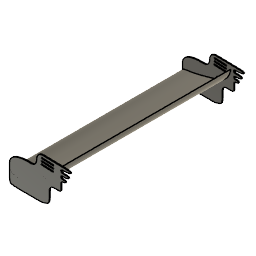
Airfoil_Design_Challenge_BITS (Autodesk Fusion 360 design; units mm, degrees)
Autodesk Fusion 360 part; units mm, degrees
(part 1 of 3)
sketch "Sketch2" plane through (0, 0, 0) normal (0, 1, 0) x (1, 0, 0)
  line L0 (0, 0) -> (212.4767, -57.0409) construction
  spline S0 degree 5 poles (212.4767, -57.0409) (212.4811, -57.0327) (212.4467, -56.9897) (212.2662, -56.8437) (211.8427, -56.5229) (211.2763, -56.0593) (210.7601, -55.5856) (210.2741, -55.0978) (209.7539, -54.5681) (209.168, -53.9856) (208.5221, -53.358) (207.8379, -52.7014) (207.1411, -52.0335) (206.4439, -51.3646) (205.7448, -50.6977) (205.0353, -50.0315) (204.304, -49.3629) (203.5422, -48.6889) (202.7475, -48.0094) (201.9215, -47.3254) (201.068, -46.6387) (200.192, -45.951) (199.2971, -45.2633) (198.3853, -44.5755) (197.4571, -43.8867) (196.5121, -43.1956) (195.5499, -42.5009) (194.5701, -41.8014) (193.573, -41.0967) (192.5596, -40.3867) (191.531, -39.6718) (190.4885, -38.9526) (189.4335, -38.2295) (188.367, -37.503) (187.2896, -36.7733) (186.2017, -36.0406) (185.1036, -35.3049) (183.9954, -34.5662) (182.8772, -33.8244) (181.7492, -33.0797) (180.6116, -32.3321) (179.4648, -31.5818) (178.3092, -30.8291) (177.1453, -30.0741) (175.9734, -29.3171) (174.7941, -28.5585) (173.6076, -27.7983) (172.4142, -27.037) (171.214, -26.2745) (170.0073, -25.5112) (168.7943, -24.7472) (167.575, -23.9826) (166.3497, -23.2178) (165.1186, -22.4528) (163.8818, -21.6879) (162.6396, -20.9232) (161.3921, -20.1589) (160.1396, -19.3954) (158.8823, -18.6326) (157.6203, -17.8709) (156.3539, -17.1105) (155.083, -16.3515) (153.808, -15.5943) (152.5288, -14.8389) (151.2457, -14.0856) (149.9587, -13.3347) (148.668, -12.5865) (147.3737, -11.8411) (146.076, -11.0988) (144.7749, -10.3599) (143.4707, -9.6246) (142.1634, -8.8933) (140.8531, -8.1661) (139.5399, -7.4433) (138.224, -6.725) (136.9055, -6.0116) (135.5843, -5.3032) (134.2607, -4.6001) (132.9347, -3.9025) (131.6065, -3.2107) (130.276, -2.5249) (128.9436, -1.8455) (127.6091, -1.1728) (126.2728, -0.5071) (124.9347, 0.1512) (123.5949, 0.8016) (122.2533, 1.4439) (120.9099, 2.0774) (119.5648, 2.7017) (118.2177, 3.3163) (116.8686, 3.9208) (115.5175, 4.5148) (114.1642, 5.0979) (112.8087, 5.6698) (111.4509, 6.2305) (110.0908, 6.7796) (108.7284, 7.3172) (107.3638, 7.8432) (105.9969, 8.3576) (104.6278, 8.8602) (103.2565, 9.3511) (101.8833, 9.83) (100.5082, 10.297) (99.1313, 10.7518) (97.7527, 11.1943) (96.3726, 11.6242) (94.991, 12.0415) (93.6081, 12.4458) (92.2239, 12.8369) (90.8384, 13.2148) (89.4519, 13.579) (88.0643, 13.9296) (86.6758, 14.2663) (85.2866, 14.5892) (83.8968, 14.8981) (82.5067, 15.1932) (81.1165, 15.4744) (79.7264, 15.7418) (78.3367, 15.9955) (76.9475, 16.2356) (75.5591, 16.4621) (74.1716, 16.6749) (72.7851, 16.8742) (71.4, 17.0599) (70.0162, 17.232) (68.6341, 17.3906) (67.2537, 17.5358) (65.8755, 17.6677) (64.4996, 17.7863) (63.1263, 17.8919) (61.7559, 17.9845) (60.3886, 18.0643) (59.0249, 18.1313) (57.6649, 18.1857) (56.309, 18.2276) (54.9573, 18.2569) (53.6102, 18.2736) (52.2679, 18.2779) (50.9307, 18.2696) (49.5988, 18.2488) (48.2726, 18.2154) (46.9524, 18.1694) (45.6385, 18.1109) (44.3312, 18.0398) (43.0308, 17.956) (41.7378, 17.8596) (40.4523, 17.7505) (39.1749, 17.6288) (37.9058, 17.4945) (36.6455, 17.3474) (35.3941, 17.1877) (34.1522, 17.0152) (32.92, 16.8299) (31.6978, 16.6317) (30.4861, 16.4207) (29.2853, 16.1966) (28.0958, 15.9595) (26.918, 15.7094) (25.7525, 15.4461) (24.5999, 15.1696) (23.4607, 14.8798) (22.3355, 14.5768) (21.2247, 14.2603) (20.1289, 13.9304) (19.0487, 13.587) (17.9846, 13.2299) (16.9373, 12.859) (15.9075, 12.4743) (14.896, 12.0756) (13.9038, 11.6629) (12.9318, 11.236) (11.9809, 10.7949) (11.052, 10.3396) (10.1459, 9.8701) (9.2635, 9.3866) (8.4059, 8.8889) (7.5744, 8.377) (6.7708, 7.8508) (5.9972, 7.3098) (5.2557, 6.754) (4.5484, 6.1836) (3.8771, 5.599) (3.2432, 5.0012) (2.6484, 4.3911) (2.0954, 3.7688) (1.5881, 3.1334) (1.1324, 2.4835) (0.7358, 1.8248) (0.4076, 1.1735) (0.1598, 0.566) (-0.0008, 0.0444) (-0.0815, -0.36) (-0.1201, -0.6567) (-0.145, -0.8932) (-0.1463, -1.2408) (-0.1178, -1.4667) (-0.1072, -1.5898) (-0.0507, -1.8099) (-0.0051, -1.9331) (0.0982, -2.1251) (0.1853, -2.2519) (0.289, -2.4175) (0.5475, -2.7065) (0.7064, -2.8823) (0.9696, -3.1172) (1.323, -3.4157) (1.6012, -3.648) (1.8666, -3.8408) (2.3156, -4.1171) (3.0047, -4.5094) (3.8866, -4.9842) (4.8656, -5.4778) (5.8455, -5.9275) (6.7856, -6.3085) (7.6894, -6.626) (8.585, -6.902) (9.5098, -7.1644) (10.4912, -7.4339) (11.5355, -7.7165) (12.6366, -8.0096) (13.7801, -8.3045) (14.9495, -8.591) (16.1317, -8.8613) (17.3214, -9.1127) (18.5188, -9.3462) (19.7275, -9.5655) (20.9531, -9.7752) (22.2012, -9.98) (23.475, -10.1832) (24.7753, -10.3861) (26.1011, -10.5891) (27.4501, -10.7914) (28.8195, -10.9921) (30.2063, -11.1904) (31.6084, -11.3859) (33.0247, -11.5791) (34.4546, -11.7708) (35.8983, -11.9624) (37.3562, -12.1554) (38.8286, -12.3512) (40.3159, -12.5513) (41.8181, -12.7565) (43.3347, -12.9675) (44.8651, -13.1845) (46.4085, -13.4076) (47.9638, -13.6368) (49.5301, -13.8718) (51.1066, -14.1126) (52.6927, -14.3591) (54.2877, -14.6112) (55.8914, -14.8691) (57.5035, -15.1329) (59.1238, -15.4028) (60.7521, -15.679) (62.3882, -15.962) (64.032, -16.2518) (65.6829, -16.5489) (67.3406, -16.8536) (69.0047, -17.166) (70.6745, -17.4866) (72.3495, -17.8154) (74.0292, -18.1525) (75.713, -18.498) (77.4005, -18.8518) (79.091, -19.2136) (80.7843, -19.5832) (82.4799, -19.9603) (84.1774, -20.3443) (85.8766, -20.7348) (87.5771, -21.1312) (89.2787, -21.5331) (90.9811, -21.94) (92.6841, -22.3512) (94.3874, -22.7663) (96.0908, -23.1849) (97.7942, -23.6065) (99.4973, -24.0306) (101.2001, -24.457) (102.9022, -24.8853) (104.6035, -25.3152) (106.3039, -25.7464) (108.0033, -26.1788) (109.7014, -26.6122) (111.398, -27.0465) (113.0931, -27.4815) (114.7865, -27.9172) (116.478, -28.3535) (118.1675, -28.7903) (119.8547, -29.2277) (121.5396, -29.6654) (123.2219, -30.1036) (124.9015, -30.5421) (126.5782, -30.981) (128.2518, -31.4202) (129.922, -31.8597) (131.5886, -32.2996) (133.2513, -32.7398) (134.9098, -33.1805) (136.5639, -33.6215) (138.2132, -34.063) (139.8575, -34.5051) (141.4964, -34.9476) (143.1296, -35.3908) (144.7568, -35.8345) (146.3777, -36.2789) (147.9922, -36.7238) (149.5999, -37.1693) (151.2005, -37.6154) (152.7937, -38.0619) (154.3793, -38.5087) (155.9568, -38.9557) (157.5259, -39.4027) (159.0863, -39.8495) (160.6374, -40.2958) (162.179, -40.7415) (163.7106, -41.1863) (165.232, -41.63) (166.7429, -42.0726) (168.2431, -42.514) (169.7326, -42.9541) (171.2113, -43.3932) (172.6792, -43.8311) (174.136, -44.268) (175.5817, -44.7038) (177.0156, -45.1382) (178.4372, -45.5712) (179.8454, -46.0021) (181.2394, -46.4304) (182.6181, -46.8558) (183.9806, -47.2777) (185.3264, -47.6961) (186.6553, -48.1109) (187.9678, -48.5227) (189.2648, -48.9323) (190.5471, -49.3404) (191.8152, -49.7475) (193.069, -50.1538) (194.3073, -50.5586) (195.5275, -50.9603) (196.7252, -51.3563) (197.8965, -51.744) (199.0375, -52.1213) (200.1469, -52.4876) (201.2255, -52.8442) (202.2787, -53.1956) (203.3138, -53.5477) (204.3365, -53.9054) (205.3477, -54.2702) (206.3402, -54.6382) (207.2946, -54.9968) (208.1849, -55.3291) (208.9927, -55.6238) (209.7156, -55.8811) (210.3847, -56.1254) (211.0537, -56.3976) (211.7317, -56.7089) (212.2101, -56.9445) (212.4199, -57.0387) (212.4722, -57.049) (212.4767, -57.0409) knots 0 0 0 0 0 0 0.0028169 0.0056338 0.0084507 0.01126761 0.01408451 0.01690141 0.01971831 0.02253521 0.02535211 0.02816901 0.03098592 0.03380282 0.03661972 0.03943662 0.04225352 0.04507042 0.04788732 0.05070423 0.05352113 0.05633803 0.05915493 0.06197183 0.06478873 0.06760563 0.07042254 0.07323944 0.07605634 0.07887324 0.08169014 0.08450704 0.08732394 0.09014085 0.09295775 0.09577465 0.09859155 0.10140845 0.10422535 0.10704225 0.10985915 0.11267606 0.11549296 0.11830986 0.12112676 0.12394366 0.12676056 0.12957746 0.13239437 0.13521127 0.13802817 0.14084507 0.14366197 0.14647887 0.14929577 0.15211268 0.15492958 0.15774648 0.16056338 0.16338028 0.16619718 0.16901408 0.17183099 0.17464789 0.17746479 0.18028169 0.18309859 0.18591549 0.18873239 0.1915493 0.1943662 0.1971831 0.2 0.2028169 0.2056338 0.2084507 0.21126761 0.21408451 0.21690141 0.21971831 0.22253521 0.22535211 0.22816901 0.23098592 0.23380282 0.23661972 0.23943662 0.24225352 0.24507042 0.24788732 0.25070423 0.25352113 0.25633803 0.25915493 0.26197183 0.26478873 0.26760563 0.27042254 0.27323944 0.27605634 0.27887324 0.28169014 0.28450704 0.28732394 0.29014085 0.29295775 0.29577465 0.29859155 0.30140845 0.30422535 0.30704225 0.30985915 0.31267606 0.31549296 0.31830986 0.32112676 0.32394366 0.32676056 0.32957746 0.33239437 0.33521127 0.33802817 0.34084507 0.34366197 0.34647887 0.34929577 0.35211268 0.35492958 0.35774648 0.36056338 0.36338028 0.36619718 0.36901408 0.37183099 0.37464789 0.37746479 0.38028169 0.38309859 0.38591549 0.38873239 0.3915493 0.3943662 0.3971831 0.4 0.4028169 0.4056338 0.4084507 0.41126761 0.41408451 0.41690141 0.41971831 0.42253521 0.42535211 0.42816901 0.43098592 0.43380282 0.43661972 0.43943662 0.44225352 0.44507042 0.44788732 0.45070423 0.45352113 0.45633803 0.45915493 0.46197183 0.46478873 0.46760563 0.47042254 0.47323944 0.47605634 0.47887324 0.48169014 0.48450704 0.48732394 0.49014085 0.49295775 0.49577465 0.49859155 0.50140845 0.50422535 0.50704225 0.50985915 0.51267606 0.51549296 0.51830986 0.52112676 0.52394366 0.52676056 0.52957746 0.53239437 0.53521127 0.53802817 0.54084507 0.54366197 0.54647887 0.54929577 0.55211268 0.55492958 0.55774648 0.56056338 0.56338028 0.56619718 0.56901408 0.57183099 0.57464789 0.57746479 0.58028169 0.58309859 0.58591549 0.58873239 0.5915493 0.5943662 0.5971831 0.6 0.6028169 0.6056338 0.6084507 0.61126761 0.61408451 0.61690141 0.61971831 0.62253521 0.62535211 0.62816901 0.63098592 0.63380282 0.63661972 0.63943662 0.64225352 0.64507042 0.64788732 0.65070423 0.65352113 0.65633803 0.65915493 0.66197183 0.66478873 0.66760563 0.67042254 0.67323944 0.67605634 0.67887324 0.68169014 0.68450704 0.68732394 0.69014085 0.69295775 0.69577465 0.69859155 0.70140845 0.70422535 0.70704225 0.70985915 0.71267606 0.71549296 0.71830986 0.72112676 0.72394366 0.72676056 0.72957746 0.73239437 0.73521127 0.73802817 0.74084507 0.74366197 0.74647887 0.74929577 0.75211268 0.75492958 0.75774648 0.76056338 0.76338028 0.76619718 0.76901408 0.77183099 0.77464789 0.77746479 0.78028169 0.78309859 0.78591549 0.78873239 0.7915493 0.7943662 0.7971831 0.8 0.8028169 0.8056338 0.8084507 0.81126761 0.81408451 0.81690141 0.81971831 0.82253521 0.82535211 0.82816901 0.83098592 0.83380282 0.83661972 0.83943662 0.84225352 0.84507042 0.84788732 0.85070423 0.85352113 0.85633803 0.85915493 0.86197183 0.86478873 0.86760563 0.87042254 0.87323944 0.87605634 0.87887324 0.88169014 0.88450704 0.88732394 0.89014085 0.89295775 0.89577465 0.89859155 0.90140845 0.90422535 0.90704225 0.90985915 0.91267606 0.91549296 0.91830986 0.92112676 0.92394366 0.92676056 0.92957746 0.93239437 0.93521127 0.93802817 0.94084507 0.94366197 0.94647887 0.94929577 0.95211268 0.95492958 0.95774648 0.96056338 0.96338028 0.96619718 0.96901408 0.97183099 0.97464789 0.97746479 0.98028169 0.98309859 0.98591549 0.98873239 0.9915493 0.9943662 0.9971831 1 1 1 1 1 1
  line L1 (212.4767, -57.0409) -> (212.4767, -65.0409) construction
  line L2 (212.4767, -65.0409) -> (207.4767, -65.0409) construction
  line L3 (207.4767, -65.0409) -> (293.6674, -148.5343) construction
  spline S1 degree 5 poles (293.6674, -148.5343) (293.6768, -148.4864) (293.6956, -148.3905) (293.7231, -148.2462) (293.7587, -148.0528) (293.8015, -147.8097) (293.8425, -147.5655) (293.8817, -147.321) (293.919, -147.0771) (293.9544, -146.8358) (293.9879, -146.5991) (294.0191, -146.3692) (294.0478, -146.1475) (294.0735, -145.9347) (294.0954, -145.7298) (294.1126, -145.5303) (294.1241, -145.3328) (294.1293, -145.1341) (294.128, -144.9318) (294.1207, -144.7252) (294.1085, -144.5151) (294.093, -144.3031) (294.0755, -144.0911) (294.0574, -143.8807) (294.0397, -143.6731) (294.0228, -143.4686) (294.007, -143.2671) (293.9917, -143.0681) (293.976, -142.8708) (293.9584, -142.674) (293.9376, -142.4768) (293.9125, -142.2784) (293.8827, -142.0782) (293.8491, -141.8763) (293.8131, -141.6731) (293.7762, -141.4693) (293.7399, -141.2654) (293.7045, -141.0618) (293.6698, -140.8583) (293.635, -140.6548) (293.5992, -140.4513) (293.5615, -140.2476) (293.5218, -140.044) (293.4801, -139.8409) (293.437, -139.6388) (293.3934, -139.4383) (293.3501, -139.2401) (293.3083, -139.0447) (293.2688, -138.8526) (293.2322, -138.6639) (293.1987, -138.4787) (293.1676, -138.2963) (293.138, -138.116) (293.1084, -137.9368) (293.0773, -137.7575) (293.0435, -137.577) (293.0057, -137.3943) (292.9634, -137.2086) (292.9165, -137.0197) (292.8656, -136.8278) (292.812, -136.6337) (292.7573, -136.4384) (292.7032, -136.2432) (292.6508, -136.0487) (292.6006, -135.8552) (292.5524, -135.6626) (292.5058, -135.4705) (292.4599, -135.2784) (292.4141, -135.0858) (292.3676, -134.8923) (292.3198, -134.6977) (292.2703, -134.5018) (292.2189, -134.3047) (292.1654, -134.1061) (292.1102, -133.9064) (292.0535, -133.7056) (291.9957, -133.504) (291.9372, -133.3019) (291.8786, -133.0998) (291.8202, -132.898) (291.7624, -132.6969) (291.7053, -132.4967) (291.6489, -132.2975) (291.593, -132.0993) (291.5373, -131.902) (291.4815, -131.7052) (291.4251, -131.5087) (291.368, -131.3122) (291.3097, -131.1154) (291.2502, -130.9181) (291.1895, -130.7202) (291.1276, -130.5216) (291.0648, -130.3225) (291.0015, -130.1231) (290.938, -129.9237) (290.8745, -129.7244) (290.8114, -129.5255) (290.7487, -129.3268) (290.6864, -129.1284) (290.6243, -128.9301) (290.5624, -128.7318) (290.5002, -128.5334) (290.4376, -128.3347) (290.3743, -128.1355) (290.31, -127.9358) (290.2447, -127.7355) (290.1784, -127.5346) (290.1113, -127.3332) (290.0434, -127.1314) (289.9749, -126.9291) (289.9058, -126.7263) (289.8362, -126.523) (289.766, -126.3193) (289.6952, -126.1149) (289.6237, -125.91) (289.5515, -125.7046) (289.4786, -125.4988) (289.4049, -125.2925) (289.3305, -125.0859) (289.2555, -124.879) (289.1798, -124.6716) (289.1035, -124.4638) (289.0266, -124.2553) (288.9491, -124.0462) (288.8709, -123.8365) (288.7921, -123.6263) (288.7126, -123.4158) (288.6325, -123.2054) (288.5517, -122.9951) (288.4706, -122.7851) (288.3893, -122.5756) (288.3084, -122.3664) (288.228, -122.1576) (288.1482, -121.949) (288.069, -121.7404) (287.9898, -121.5316) (287.9099, -121.3224) (287.8287, -121.1126) (287.7458, -120.902) (287.6607, -120.6905) (287.5738, -120.4782) (287.4854, -120.2651) (287.3962, -120.0512) (287.3067, -119.8367) (287.2173, -119.6217) (287.1282, -119.4062) (287.0391, -119.1904) (286.9498, -118.9742) (286.86, -118.7578) (286.7693, -118.5411) (286.6776, -118.3242) (286.5848, -118.1069) (286.4909, -117.8894) (286.3959, -117.6716) (286.3001, -117.4534) (286.2035, -117.235) (286.1065, -117.0164) (286.0092, -116.7976) (285.9116, -116.5786) (285.8139, -116.3594) (285.7159, -116.1401) (285.6173, -115.9203) (285.5177, -115.7) (285.417, -115.4789) (285.3146, -115.257) (285.2107, -115.0343) (285.1053, -114.8107) (284.9989, -114.5866) (284.8919, -114.3621) (284.7847, -114.1374) (284.6779, -113.9129) (284.5716, -113.6886) (284.4657, -113.4646) (284.3599, -113.2408) (284.254, -113.017) (284.1475, -112.7932) (284.0402, -112.5692) (283.9317, -112.3449) (283.8221, -112.1202) (283.7113, -111.895) (283.5995, -111.6695) (283.4868, -111.4436) (283.3734, -111.2175) (283.2596, -110.9912) (283.1454, -110.765) (283.0311, -110.539) (282.9167, -110.3134) (282.8023, -110.0881) (282.6877, -109.8632) (282.5728, -109.6386) (282.4573, -109.4141) (282.341, -109.1897) (282.2237, -108.9651) (282.1053, -108.7403) (281.9857, -108.5153) (281.8652, -108.2903) (281.7439, -108.0653) (281.6219, -107.8405) (281.4996, -107.6161) (281.377, -107.3922) (281.2542, -107.1688) (281.1312, -106.9459) (281.0078, -106.7234) (280.8841, -106.5012) (280.76, -106.2793) (280.6355, -106.0577) (280.5104, -105.8363) (280.3849, -105.6151) (280.259, -105.3941) (280.1327, -105.1735) (280.006, -104.9531) (279.8791, -104.7331) (279.7518, -104.5133) (279.6242, -104.2939) (279.4963, -104.0747) (279.3681, -103.8557) (279.2396, -103.637) (279.1107, -103.4185) (278.9817, -103.2002) (278.8523, -102.9821) (278.7227, -102.7641) (278.5929, -102.5464) (278.4627, -102.3289) (278.3322, -102.1117) (278.2013, -101.8948) (278.0699, -101.6783) (277.9379, -101.4623) (277.8053, -101.2469) (277.672, -101.0319) (277.5381, -100.8175) (277.4034, -100.6036) (277.2682, -100.3902) (277.1323, -100.1774) (276.9957, -99.965) (276.8586, -99.7532) (276.7208, -99.5419) (276.5825, -99.331) (276.4435, -99.1207) (276.304, -98.9108) (276.1641, -98.7013) (276.0238, -98.4921) (275.8833, -98.2831) (275.7426, -98.0742) (275.6018, -97.8654) (275.461, -97.6565) (275.3202, -97.4478) (275.1793, -97.2391) (275.0382, -97.0305) (274.897, -96.8221) (274.7554, -96.6139) (274.6134, -96.4061) (274.4711, -96.1986) (274.3283, -95.9914) (274.1851, -95.7847) (274.0415, -95.5782) (273.8974, -95.3722) (273.7529, -95.1666) (273.6079, -94.9613) (273.4623, -94.7566) (273.3161, -94.5524) (273.1693, -94.3487) (273.0219, -94.1455) (272.8739, -93.9428) (272.7253, -93.7407) (272.5762, -93.539) (272.4265, -93.3378) (272.2764, -93.137) (272.1258, -92.9365) (271.9748, -92.7365) (271.8234, -92.5368) (271.6715, -92.3375) (271.5192, -92.1387) (271.3664, -91.9403) (271.2131, -91.7423) (271.0593, -91.5448) (270.905, -91.3477) (270.7502, -91.151) (270.5949, -90.9547) (270.4391, -90.7588) (270.2828, -90.5633) (270.1261, -90.3683) (269.9689, -90.1736) (269.8113, -89.9794) (269.6533, -89.7855) (269.495, -89.592) (269.3364, -89.3989) (269.1774, -89.206) (269.0183, -89.0134) (268.8588, -88.821) (268.699, -88.6289) (268.539, -88.437) (268.3786, -88.2455) (268.2177, -88.0543) (268.0564, -87.8636) (267.8947, -87.6734) (267.7323, -87.4836) (267.5695, -87.2944) (267.4061, -87.1057) (267.2421, -86.9175) (267.0776, -86.7297) (266.9126, -86.5424) (266.747, -86.3556) (266.5809, -86.1692) (266.4144, -85.9833) (266.2473, -85.7978) (266.0798, -85.6129) (265.9118, -85.4284) (265.7434, -85.2445) (265.5744, -85.0611) (265.405, -84.8782) (265.2351, -84.6958) (265.0647, -84.5138) (264.8938, -84.3324) (264.7224, -84.1513) (264.5506, -83.9707) (264.3783, -83.7904) (264.2056, -83.6106) (264.0325, -83.4311) (263.8588, -83.252) (263.6848, -83.0735) (263.5102, -82.8954) (263.3351, -82.7179) (263.1595, -82.541) (262.9834, -82.3648) (262.8066, -82.1891) (262.6292, -82.0141) (262.4512, -81.8398) (262.2725, -81.666) (262.0931, -81.4928) (261.9132, -81.3202) (261.7327, -81.1482) (261.5516, -80.9767) (261.37, -80.8059) (261.1879, -80.6356) (261.0053, -80.4659) (260.8221, -80.2969) (260.6384, -80.1284) (260.4541, -79.9606) (260.2692, -79.7934) (260.0837, -79.6268) (259.8976, -79.4607) (259.7111, -79.295) (259.5241, -79.1298) (259.3367, -78.965) (259.149, -78.8006) (258.9609, -78.6365) (258.7724, -78.4729) (258.5835, -78.3099) (258.3939, -78.1475) (258.2038, -77.9859) (258.013, -77.825) (257.8216, -77.6649) (257.6296, -77.5054) (257.4371, -77.3465) (257.2441, -77.188) (257.0507, -77.03) (256.857, -76.8723) (256.6629, -76.715) (256.4684, -76.5581) (256.2734, -76.4017) (256.078, -76.2458) (255.882, -76.0904) (255.6856, -75.9356) (255.4888, -75.7814) (255.2915, -75.6276) (255.0939, -75.4743) (254.896, -75.3214) (254.6978, -75.1689) (254.4992, -75.0167) (254.3003, -74.865) (254.1011, -74.7138) (253.9013, -74.563) (253.7011, -74.4128) (253.5004, -74.2631) (253.2991, -74.114) (253.0973, -73.9654) (252.895, -73.8174) (252.6923, -73.67) (252.4891, -73.5231) (252.2854, -73.3769) (252.0812, -73.2312) (251.8765, -73.0861) (251.6714, -72.9415) (251.4657, -72.7976) (251.2596, -72.6543) (251.0529, -72.5116) (250.8457, -72.3696) (250.6379, -72.2282) (250.4296, -72.0875) (250.2207, -71.9475) (250.0113, -71.8081) (249.8014, -71.6694) (249.591, -71.5313) (249.3801, -71.3938) (249.1687, -71.2569) (248.9569, -71.1206) (248.7445, -70.9849) (248.5316, -70.8498) (248.3182, -70.7155) (248.1042, -70.5818) (247.8897, -70.4489) (247.6747, -70.3166) (247.4592, -70.1849) (247.2432, -70.0537) (247.0269, -69.9231) (246.8103, -69.7928) (246.5933, -69.663) (246.3759, -69.5337) (246.1581, -69.405) (245.9398, -69.2769) (245.7209, -69.1496) (245.5014, -69.0231) (245.2812, -68.8974) (245.0605, -68.7725) (244.8392, -68.6483) (244.6174, -68.5248) (244.3952, -68.4019) (244.1725, -68.2796) (243.9494, -68.1579) (243.7259, -68.0368) (243.5018, -67.9165) (243.2771, -67.7968) (243.0517, -67.678) (242.8256, -67.5602) (242.5988, -67.4432) (242.3714, -67.3272) (242.1435, -67.212) (241.9151, -67.0977) (241.6862, -66.9842) (241.4569, -66.8714) (241.2271, -66.7591) (240.9968, -66.6473) (240.7659, -66.5359) (240.5343, -66.4248) (240.3021, -66.3142) (240.0694, -66.2041) (239.8364, -66.0947) (239.6032, -65.9864) (239.3702, -65.8792) (239.1374, -65.7735) (238.9053, -65.6693) (238.6737, -65.5665) (238.443, -65.4651) (238.2131, -65.3648) (237.984, -65.2656) (237.756, -65.1674) (237.529, -65.0703) (237.3033, -64.9748) (237.0791, -64.8811) (236.8564, -64.7896) (236.6354, -64.7008) (236.4161, -64.6146) (236.1985, -64.531) (235.9825, -64.4498) (235.7678, -64.3704) (235.5542, -64.2925) (235.3415, -64.2156) (235.1294, -64.1395) (234.9177, -64.064) (234.7062, -63.9892) (234.4949, -63.9151) (234.2838, -63.8418) (234.0728, -63.7694) (233.8622, -63.6979) (233.6522, -63.6276) (233.4431, -63.5585) (233.235, -63.4907) (233.028, -63.4243) (232.8222, -63.3596) (232.6176, -63.2964) (232.4141, -63.235) (232.2116, -63.1753) (232.0101, -63.117) (231.8095, -63.0601) (231.6095, -63.0043) (231.4102, -62.9493) (231.2114, -62.8948) (231.0131, -62.8404) (230.8151, -62.786) (230.6174, -62.7315) (230.4202, -62.6773) (230.2237, -62.6237) (230.028, -62.5718) (229.8335, -62.5222) (229.6403, -62.4756) (229.4483, -62.4318) (229.2571, -62.3902) (229.0665, -62.3499) (228.8759, -62.3096) (228.6851, -62.2686) (228.4939, -62.2268) (228.3025, -62.1845) (228.1113, -62.1424) (227.9205, -62.1012) (227.7304, -62.0617) (227.5411, -62.024) (227.3528, -61.9882) (227.1654, -61.9541) (226.9787, -61.9214) (226.7925, -61.8895) (226.6064, -61.8578) (226.4202, -61.8259) (226.2337, -61.7936) (226.0468, -61.761) (225.8598, -61.7288) (225.6729, -61.6976) (225.4864, -61.668) (225.3005, -61.6404) (225.1153, -61.6152) (224.931, -61.5922) (224.7475, -61.5712) (224.5646, -61.5517) (224.382, -61.533) (224.1994, -61.5145) (224.0165, -61.4957) (223.8333, -61.4764) (223.6499, -61.4569) (223.4666, -61.4377) (223.2838, -61.4192) (223.1021, -61.4018) (222.9218, -61.3856) (222.7434, -61.3706) (222.5671, -61.3569) (222.3932, -61.3447) (222.2216, -61.3344) (222.0522, -61.3265) (221.8843, -61.321) (221.7174, -61.3174) (221.5506, -61.3143) (221.3829, -61.3103) (221.2139, -61.304) (221.0433, -61.2952) (220.8716, -61.2847) (220.6996, -61.2738) (220.5283, -61.2642) (220.3584, -61.2574) (220.1906, -61.2545) (220.0253, -61.2561) (219.8625, -61.2618) (219.7019, -61.2701) (219.5426, -61.2788) (219.3838, -61.286) (219.225, -61.2911) (219.0656, -61.2949) (218.9057, -61.2989) (218.7451, -61.3043) (218.5842, -61.3117) (218.4233, -61.3205) (218.2626, -61.3297) (218.1019, -61.3387) (217.9411, -61.3473) (217.7796, -61.3561) (217.6171, -61.3655) (217.4538, -61.3758) (217.2905, -61.3871) (217.128, -61.3995) (216.9672, -61.4129) (216.8082, -61.428) (216.6511, -61.4451) (216.4953, -61.4648) (216.3406, -61.4868) (216.1865, -61.51) (216.0328, -61.5334) (215.8792, -61.5559) (215.7256, -61.5777) (215.5716, -61.5998) (215.4172, -61.6232) (215.2621, -61.6487) (215.1063, -61.6757) (214.9498, -61.7034) (214.7928, -61.731) (214.6356, -61.7583) (214.4788, -61.786) (214.3228, -61.815) (214.1682, -61.846) (214.0153, -61.8796) (213.8644, -61.9156) (213.7155, -61.9537) (213.5684, -61.9931) (213.4224, -62.033) (213.277, -62.0726) (213.1313, -62.1114) (212.9852, -62.1493) (212.8384, -62.1867) (212.6912, -62.2241) (212.5441, -62.2616) (212.398, -62.2998) (212.2537, -62.3389) (212.1118, -62.3794) (211.9722, -62.4221) (211.8346, -62.4676) (211.6985, -62.5164) (211.5633, -62.568) (211.4284, -62.6218) (211.2932, -62.6766) (211.157, -62.7316) (211.0193, -62.7859) (210.8798, -62.8396) (210.7392, -62.894) (210.5993, -62.9518) (210.4613, -63.0152) (210.3258, -63.0848) (210.1913, -63.1581) (210.0554, -63.2311) (209.916, -63.3002) (209.773, -63.3649) (209.6282, -63.428) (209.4841, -63.4934) (209.3426, -63.5641) (209.2034, -63.6398) (209.0654, -63.7186) (208.9272, -63.7981) (208.7894, -63.8774) (208.6546, -63.9579) (208.5258, -64.0418) (208.4054, -64.1312) (208.2938, -64.227) (208.1892, -64.3286) (208.089, -64.4344) (207.99, -64.5411) (207.8892, -64.6451) (207.7852, -64.744) (207.6789, -64.8386) (207.5744, -64.9339) (207.4764, -65.0358) (207.3881, -65.1484) (207.3093, -65.2708) (207.2384, -65.4001) (207.1749, -65.5326) (207.1218, -65.6678) (207.0847, -65.8067) (207.0685, -65.9497) (207.0749, -66.0939) (207.1017, -66.2337) (207.1462, -66.3645) (207.2086, -66.4863) (207.2932, -66.6055) (207.4049, -66.7308) (207.5469, -66.8691) (207.7174, -67.0225) (207.911, -67.1883) (208.1201, -67.3615) (208.3363, -67.5358) (208.5523, -67.7052) (208.7635, -67.8661) (208.9687, -68.0175) (209.1688, -68.1608) (209.3666, -68.2982) (209.5652, -68.4326) (209.7673, -68.5666) (209.9742, -68.7015) (210.1861, -68.8373) (210.402, -68.9736) (210.6206, -69.1092) (210.8404, -69.243) (211.0603, -69.3743) (211.2799, -69.5027) (211.4994, -69.6285) (211.7189, -69.7522) (211.9392, -69.8742) (212.1608, -69.9951) (212.3839, -70.1152) (212.6087, -70.2344) (212.8349, -70.3527) (213.0623, -70.4699) (213.2907, -70.5857) (213.5198, -70.6999) (213.7495, -70.8127) (213.9797, -70.9244) (214.2104, -71.0351) (214.4418, -71.1453) (214.6737, -71.2551) (214.9062, -71.3648) (215.1392, -71.4742) (215.3725, -71.5831) (215.6059, -71.6912) (215.8391, -71.7983) (216.0718, -71.9039) (216.304, -72.0078) (216.5355, -72.1101) (216.7662, -72.2106) (216.996, -72.3096) (217.225, -72.4071) (217.4532, -72.5034) (217.6809, -72.5988) (217.908, -72.6934) (218.1348, -72.7876) (218.3614, -72.8815) (218.5878, -72.9752) (218.8141, -73.0687) (219.0401, -73.1616) (219.2656, -73.2537) (219.4905, -73.3447) (219.7146, -73.4343) (219.9379, -73.5225) (220.1602, -73.6091) (220.3817, -73.6946) (220.6025, -73.7791) (220.8229, -73.8629) (221.0428, -73.9463) (221.2625, -74.0296) (221.4819, -74.1126) (221.701, -74.1955) (221.9198, -74.278) (222.1382, -74.3601) (222.3562, -74.4417) (222.5735, -74.5226) (222.7903, -74.6029) (223.0064, -74.6825) (223.2218, -74.7614) (223.4366, -74.8399) (223.6509, -74.9179) (223.8649, -74.9956) (224.0788, -75.0731) (224.2926, -75.1507) (224.5065, -75.2283) (224.7206, -75.3062) (224.9347, -75.3843) (225.1489, -75.4626) (225.363, -75.5412) (225.577, -75.6198) (225.791, -75.6985) (226.0049, -75.7769) (226.2188, -75.855) (226.4328, -75.9328) (226.6468, -76.0102) (226.861, -76.0875) (227.0752, -76.1651) (227.2895, -76.2431) (227.5037, -76.3219) (227.7177, -76.4015) (227.9315, -76.4815) (228.145, -76.5617) (228.3579, -76.6414) (228.5703, -76.7203) (228.7821, -76.798) (228.9934, -76.8746) (229.2042, -76.9506) (229.4147, -77.0265) (229.625, -77.1028) (229.8353, -77.1797) (230.0456, -77.2574) (230.2559, -77.3354) (230.4662, -77.4134) (230.6765, -77.4909) (230.8868, -77.5676) (231.0972, -77.6438) (231.3078, -77.7196) (231.5187, -77.7958) (231.73, -77.8728) (231.9417, -77.951) (232.1539, -78.0305) (232.3664, -78.1112) (232.5793, -78.1925) (232.7922, -78.274) (233.0052, -78.3555) (233.2181, -78.4365) (233.4308, -78.517) (233.6433, -78.5971) (233.8556, -78.6769) (234.0676, -78.7567) (234.2796, -78.8367) (234.4915, -78.9171) (234.7037, -78.9982) (234.9161, -79.08) (235.1289, -79.1627) (235.3422, -79.2462) (235.556, -79.3306) (235.7702, -79.4156) (235.9847, -79.5011) (236.1996, -79.5871) (236.4148, -79.6735) (236.6304, -79.7605) (236.8464, -79.8482) (237.0628, -79.9367) (237.2797, -80.0261) (237.4971, -80.1164) (237.7148, -80.2073) (237.9327, -80.2987) (238.1507, -80.3901) (238.3686, -80.4813) (238.5865, -80.5722) (238.8042, -80.6629) (239.022, -80.7535) (239.2397, -80.8443) (239.4577, -80.9357) (239.6759, -81.0279) (239.8945, -81.1211) (240.1134, -81.2154) (240.3326, -81.3109) (240.5522, -81.4073) (240.7719, -81.5047) (240.9919, -81.6027) (241.212, -81.7014) (241.4323, -81.8006) (241.6528, -81.9001) (241.8735, -82) (242.0944, -82.1002) (242.3157, -82.201) (242.5373, -82.3024) (242.7595, -82.4048) (242.9822, -82.5084) (243.2056, -82.6132) (243.4297, -82.7194) (243.6544, -82.8269) (243.8798, -82.9356) (244.1059, -83.0452) (244.3324, -83.1556) (244.5594, -83.2665) (244.7866, -83.3778) (245.0138, -83.4892) (245.241, -83.6007) (245.4679, -83.7123) (245.6943, -83.8239) (245.9204, -83.9357) (246.1462, -84.0478) (246.3717, -84.1606) (246.5972, -84.2741) (246.8227, -84.3885) (247.0484, -84.5041) (247.2742, -84.6208) (247.5002, -84.7386) (247.7261, -84.8572) (247.9519, -84.9764) (248.1773, -85.0961) (248.4023, -85.2161) (248.6268, -85.3364) (248.8509, -85.4568) (249.0745, -85.5776) (249.2978, -85.6986) (249.5208, -85.82) (249.7436, -85.9418) (249.9662, -86.0641) (250.1886, -86.1868) (250.4107, -86.31) (250.6326, -86.4336) (250.8542, -86.5577) (251.0755, -86.6821) (251.2964, -86.807) (251.517, -86.9323) (251.7373, -87.0579) (251.9571, -87.184) (252.1766, -87.3106) (252.3957, -87.4377) (252.6144, -87.5653) (252.8327, -87.6934) (253.0504, -87.8222) (253.2678, -87.9515) (253.4847, -88.0814) (253.7011, -88.2119) (253.9171, -88.3429) (254.1328, -88.4745) (254.3481, -88.6065) (254.563, -88.739) (254.7775, -88.8719) (254.9916, -89.0054) (255.2052, -89.1395) (255.4184, -89.2741) (255.6311, -89.4094) (255.8433, -89.5453) (256.055, -89.6818) (256.2664, -89.8187) (256.4775, -89.9559) (256.6884, -90.0934) (256.8992, -90.2311) (257.1098, -90.3689) (257.3202, -90.507) (257.5304, -90.6455) (257.7402, -90.7843) (257.9496, -90.9237) (258.1585, -91.0637) (258.3669, -91.2042) (258.5748, -91.3454) (258.7823, -91.4871) (258.9894, -91.6294) (259.1961, -91.772) (259.4025, -91.915) (259.6086, -92.0585) (259.8142, -92.2023) (260.0195, -92.3467) (260.2244, -92.4916) (260.4287, -92.637) (260.6326, -92.7831) (260.836, -92.9298) (261.0388, -93.077) (261.2412, -93.2249) (261.4431, -93.3732) (261.6446, -93.5221) (261.8457, -93.6714) (262.0463, -93.8213) (262.2466, -93.9716) (262.4464, -94.1224) (262.6458, -94.2737) (262.8449, -94.4254) (263.0435, -94.5777) (263.2416, -94.7304) (263.4394, -94.8836) (263.6367, -95.0373) (263.8336, -95.1915) (264.0301, -95.3461) (264.2261, -95.5013) (264.4216, -95.657) (264.6167, -95.8133) (264.8113, -95.97) (265.0055, -96.1273) (265.1992, -96.2851) (265.3925, -96.4433) (265.5854, -96.6021) (265.7778, -96.7613) (265.9698, -96.9209) (266.1614, -97.0811) (266.3525, -97.2417) (266.5431, -97.4029) (266.7332, -97.5647) (266.9229, -97.727) (267.1121, -97.8898) (267.3008, -98.0532) (267.489, -98.217) (267.6769, -98.3812) (267.8644, -98.5457) (268.0516, -98.7106) (268.2385, -98.8757) (268.425, -99.0411) (268.6112, -99.2069) (268.7971, -99.3731) (268.9826, -99.5397) (269.1677, -99.7068) (269.3524, -99.8744) (269.5367, -100.0424) (269.7205, -100.211) (269.9039, -100.38) (270.0869, -100.5495) (270.2693, -100.7194) (270.4512, -100.89) (270.6325, -101.0612) (270.813, -101.2331) (270.9929, -101.4058) (271.1719, -101.5793) (271.3503, -101.7536) (271.528, -101.9285) (271.705, -102.1041) (271.8815, -102.2801) (272.0576, -102.4566) (272.2331, -102.6336) (272.4081, -102.811) (272.5826, -102.9889) (272.7566, -103.1673) (272.93, -103.3465) (273.1027, -103.5262) (273.275, -103.7066) (273.4467, -103.8875) (273.6181, -104.0688) (273.7891, -104.2503) (273.96, -104.432) (274.1305, -104.6139) (274.3009, -104.796) (274.4708, -104.9784) (274.6403, -105.1613) (274.8092, -105.3448) (274.9774, -105.529) (275.1449, -105.714) (275.3117, -105.8997) (275.4778, -106.086) (275.6434, -106.2729) (275.8084, -106.4602) (275.9729, -106.648) (276.1369, -106.8361) (276.3005, -107.0247) (276.4635, -107.2137) (276.6261, -107.4032) (276.7881, -107.5933) (276.9495, -107.784) (277.1105, -107.9752) (277.2709, -108.1669) (277.4308, -108.3591) (277.5903, -108.5517) (277.7492, -108.7447) (277.9075, -108.9381) (278.0653, -109.132) (278.2225, -109.3264) (278.379, -109.5216) (278.5348, -109.7174) (278.6898, -109.9139) (278.8441, -110.1111) (278.9978, -110.309) (279.1509, -110.5074) (279.3034, -110.7062) (279.4553, -110.9056) (279.6067, -111.1053) (279.7574, -111.3056) (279.9075, -111.5064) (280.057, -111.7078) (280.2056, -111.9098) (280.3536, -112.1125) (280.5008, -112.3158) (280.6473, -112.5198) (280.7932, -112.7243) (280.9384, -112.9294) (281.0831, -113.1349) (281.2272, -113.3409) (281.3706, -113.5475) (281.5132, -113.7547) (281.655, -113.9626) (281.7959, -114.1714) (281.9359, -114.381) (282.0748, -114.5915) (282.2128, -114.8028) (282.3498, -115.015) (282.4858, -115.2278) (282.621, -115.4414) (282.7553, -115.6556) (282.8888, -115.8705) (283.0214, -116.086) (283.1531, -116.3021) (283.284, -116.519) (283.4141, -116.7365) (283.5433, -116.9547) (283.6716, -117.1736) (283.7991, -117.3931) (283.9259, -117.6133) (284.0519, -117.8341) (284.1771, -118.0555) (284.3017, -118.2774) (284.4257, -118.4998) (284.549, -118.7225) (284.6718, -118.9457) (284.7939, -119.1693) (284.9156, -119.3932) (285.0367, -119.6176) (285.1574, -119.8424) (285.2775, -120.0676) (285.3972, -120.2934) (285.5163, -120.5197) (285.6347, -120.7466) (285.7525, -120.9739) (285.8695, -121.2015) (285.9856, -121.4295) (286.1006, -121.6577) (286.2146, -121.8859) (286.3274, -122.1142) (286.4391, -122.3425) (286.5497, -122.5707) (286.6591, -122.7989) (286.7675, -123.0269) (286.875, -123.2548) (286.9816, -123.4827) (287.0877, -123.7106) (287.1932, -123.9383) (287.2983, -124.1661) (287.4029, -124.3937) (287.5071, -124.6212) (287.6107, -124.8483) (287.7134, -125.075) (287.8152, -125.301) (287.9158, -125.5264) (288.0151, -125.7509) (288.1131, -125.9746) (288.21, -126.1975) (288.3059, -126.4197) (288.4008, -126.6412) (288.4947, -126.8621) (288.5877, -127.0823) (288.6795, -127.3017) (288.7701, -127.5204) (288.8592, -127.7381) (288.9468, -127.9549) (289.0331, -128.1709) (289.1181, -128.3861) (289.2023, -128.6008) (289.2859, -128.815) (289.3693, -129.029) (289.4524, -129.2427) (289.5351, -129.4561) (289.6172, -129.669) (289.6983, -129.8812) (289.7781, -130.0925) (289.8563, -130.3029) (289.9328, -130.5122) (290.0076, -130.7206) (290.0808, -130.9283) (290.1527, -131.1353) (290.2239, -131.3419) (290.2948, -131.5483) (290.366, -131.7547) (290.4381, -131.9612) (290.5112, -132.168) (290.585, -132.3748) (290.659, -132.5815) (290.7322, -132.7877) (290.8037, -132.9932) (290.873, -133.1976) (290.94, -133.4009) (291.0051, -133.6031) (291.069, -133.8043) (291.1326, -134.0049) (291.1961, -134.2049) (291.2595, -134.4046) (291.3219, -134.604) (291.3826, -134.8033) (291.4413, -135.0027) (291.4983, -135.2026) (291.5554, -135.4038) (291.6149, -135.6071) (291.6791, -135.8132) (291.7492, -136.0222) (291.8253, -136.234) (291.9049, -136.4474) (291.9846, -136.6608) (292.0608, -136.8729) (292.1306, -137.0825) (292.1925, -137.289) (292.2474, -137.4931) (292.2977, -137.6959) (292.3464, -137.8987) (292.3964, -138.1028) (292.4498, -138.3088) (292.5071, -138.5166) (292.5678, -138.7257) (292.631, -138.9353) (292.6948, -139.1446) (292.7572, -139.3529) (292.8164, -139.5597) (292.8707, -139.765) (292.9193, -139.9688) (292.9626, -140.1714) (293.0025, -140.3734) (293.0418, -140.5754) (293.0831, -140.7778) (293.1282, -140.981) (293.177, -141.1843) (293.2267, -141.3864) (293.2734, -141.5861) (293.3138, -141.7822) (293.3455, -141.9747) (293.3697, -142.165) (293.39, -142.3556) (293.4109, -142.549) (293.4362, -142.746) (293.4672, -142.9448) (293.5018, -143.1403) (293.5363, -143.3274) (293.5667, -143.5028) (293.5902, -143.6681) (293.6069, -143.8324) (293.6188, -144.0084) (293.6287, -144.2082) (293.6389, -144.4396) (293.6506, -144.7017) (293.6635, -144.9864) (293.6768, -145.2819) (293.6892, -145.5751) (293.6993, -145.8542) (293.706, -146.111) (293.7091, -146.3445) (293.7088, -146.5592) (293.7058, -146.7633) (293.701, -146.9664) (293.6953, -147.1778) (293.6891, -147.4044) (293.6831, -147.6507) (293.6774, -147.9193) (293.6731, -148.1532) (293.6702, -148.3395) (293.6683, -148.4686) (293.6674, -148.5343) knots 0 0 0 0 0 0 0.00086207 0.00172414 0.00258621 0.00344828 0.00431034 0.00517241 0.00603448 0.00689655 0.00775862 0.00862069 0.00948276 0.01034483 0.0112069 0.01206897 0.01293103 0.0137931 0.01465517 0.01551724 0.01637931 0.01724138 0.01810345 0.01896552 0.01982759 0.02068966 0.02155172 0.02241379 0.02327586 0.02413793 0.025 0.02586207 0.02672414 0.02758621 0.02844828 0.02931034 0.03017241 0.03103448 0.03189655 0.03275862 0.03362069 0.03448276 0.03534483 0.0362069 0.03706897 0.03793103 0.0387931 0.03965517 0.04051724 0.04137931 0.04224138 0.04310345 0.04396552 0.04482759 0.04568966 0.04655172 0.04741379 0.04827586 0.04913793 0.05 0.05086207 0.05172414 0.05258621 0.05344828 0.05431034 0.05517241 0.05603448 0.05689655 0.05775862 0.05862069 0.05948276 0.06034483 0.0612069 0.06206897 0.06293103 0.0637931 0.06465517 0.06551724 0.06637931 0.06724138 0.06810345 0.06896552 0.06982759 0.07068966 0.07155172 0.07241379 0.07327586 0.07413793 0.075 0.07586207 0.07672414 0.07758621 0.07844828 0.07931034 0.08017241 0.08103448 0.08189655 0.08275862 0.08362069 0.08448276 0.08534483 0.0862069 0.08706897 0.08793103 0.0887931 0.08965517 0.09051724 0.09137931 0.09224138 0.09310345 0.09396552 0.09482759 0.09568966 0.09655172 0.09741379 0.09827586 0.09913793 0.1 0.10086207 0.10172414 0.10258621 0.10344828 0.10431034 0.10517241 0.10603448 0.10689655 0.10775862 0.10862069 0.10948276 0.11034483 0.1112069 0.11206897 0.11293103 0.1137931 0.11465517 0.11551724 0.11637931 0.11724138 0.11810345 0.11896552 0.11982759 0.12068966 0.12155172 0.12241379 0.12327586 0.12413793 0.125 0.12586207 0.12672414 0.12758621 0.12844828 0.12931034 0.13017241 0.13103448 0.13189655 0.13275862 0.13362069 0.13448276 0.13534483 0.1362069 0.13706897 0.13793103 0.1387931 0.13965517 0.14051724 0.14137931 0.14224138 0.14310345 0.14396552 0.14482759 0.14568966 0.14655172 0.14741379 0.14827586 0.14913793 0.15 0.15086207 0.15172414 0.15258621 0.15344828 0.15431034 0.15517241 0.15603448 0.15689655 0.15775862 0.15862069 0.15948276 0.16034483 0.1612069 0.16206897 0.16293103 0.1637931 0.16465517 0.16551724 0.16637931 0.16724138 0.16810345 0.16896552 0.16982759 0.17068966 0.17155172 0.17241379 0.17327586 0.17413793 0.175 0.17586207 0.17672414 0.17758621 0.17844828 0.17931034 0.18017241 0.18103448 0.18189655 0.18275862 0.18362069 0.18448276 0.18534483 0.1862069 0.18706897 0.18793103 0.1887931 0.18965517 0.19051724 0.19137931 0.19224138 0.19310345 0.19396552 0.19482759 0.19568966 0.19655172 0.19741379 0.19827586 0.19913793 0.2 0.20086207 0.20172414 0.20258621 0.20344828 0.20431034 0.20517241 0.20603448 0.20689655 0.20775862 0.20862069 0.20948276 0.21034483 0.2112069 0.21206897 0.21293103 0.2137931 0.21465517 0.21551724 0.21637931 0.21724138 0.21810345 0.21896552 0.21982759 0.22068966 0.22155172 0.22241379 0.22327586 0.22413793 0.225 0.22586207 0.22672414 0.22758621 0.22844828 0.22931034 0.23017241 0.23103448 0.23189655 0.23275862 0.23362069 0.23448276 0.23534483 0.2362069 0.23706897 0.23793103 0.2387931 0.23965517 0.24051724 0.24137931 0.24224138 0.24310345 0.24396552 0.24482759 0.24568966 0.24655172 0.24741379 0.24827586 0.24913793 0.25 0.25086207 0.25172414 0.25258621 0.25344828 0.25431034 0.25517241 0.25603448 0.25689655 0.25775862 0.25862069 0.25948276 0.26034483 0.2612069 0.26206897 0.26293103 0.2637931 0.26465517 0.26551724 0.26637931 0.26724138 0.26810345 0.26896552 0.26982759 0.27068966 0.27155172 0.27241379 0.27327586 0.27413793 0.275 0.27586207 0.27672414 0.27758621 0.27844828 0.27931034 0.28017241 0.28103448 0.28189655 0.28275862 0.28362069 0.28448276 0.28534483 0.2862069 0.28706897 0.28793103 0.2887931 0.28965517 0.29051724 0.29137931 0.29224138 0.29310345 0.29396552 0.29482759 0.29568966 0.29655172 0.29741379 0.29827586 0.29913793 0.3 0.30086207 0.30172414 0.30258621 0.30344828 0.30431034 0.30517241 0.30603448 0.30689655 0.30775862 0.30862069 0.30948276 0.31034483 0.3112069 0.31206897 0.31293103 0.3137931 0.31465517 0.31551724 0.31637931 0.31724138 0.31810345 0.31896552 0.31982759 0.32068966 0.32155172 0.32241379 0.32327586 0.32413793 0.325 0.32586207 0.32672414 0.32758621 0.32844828 0.32931034 0.33017241 0.33103448 0.33189655 0.33275862 0.33362069 0.33448276 0.33534483 0.3362069 0.33706897 0.33793103 0.3387931 0.33965517 0.34051724 0.34137931 0.34224138 0.34310345 0.34396552 0.34482759 0.34568966 0.34655172 0.34741379 0.34827586 0.34913793 0.35 0.35086207 0.35172414 0.35258621 0.35344828 0.35431034 0.35517241 0.35603448 0.35689655 0.35775862 0.35862069 0.35948276 0.36034483 0.3612069 0.36206897 0.36293103 0.3637931 0.36465517 0.36551724 0.36637931 0.36724138 0.36810345 0.36896552 0.36982759 0.37068966 0.37155172 0.37241379 0.37327586 0.37413793 0.375 0.37586207 0.37672414 0.37758621 0.37844828 0.37931034 0.38017241 0.38103448 0.38189655 0.38275862 0.38362069 0.38448276 0.38534483 0.3862069 0.38706897 0.38793103 0.3887931 0.38965517 0.39051724 0.39137931 0.39224138 0.39310345 0.39396552 0.39482759 0.39568966 0.39655172 0.39741379 0.39827586 0.39913793 0.4 0.40086207 0.40172414 0.40258621 0.40344828 0.40431034 0.40517241 0.40603448 0.40689655 0.40775862 0.40862069 0.40948276 0.41034483 0.4112069 0.41206897 0.41293103 0.4137931 0.41465517 0.41551724 0.41637931 0.41724138 0.41810345 0.41896552 0.41982759 0.42068966 0.42155172 0.42241379 0.42327586 0.42413793 0.425 0.42586207 0.42672414 0.42758621 0.42844828 0.42931034 0.43017241 0.43103448 0.43189655 0.43275862 0.43362069 0.43448276 0.43534483 0.4362069 0.43706897 0.43793103 0.4387931 0.43965517 0.44051724 0.44137931 0.44224138 0.44310345 0.44396552 0.44482759 0.44568966 0.44655172 0.44741379 0.44827586 0.44913793 0.45 0.45086207 0.45172414 0.45258621 0.45344828 0.45431034 0.45517241 0.45603448 0.45689655 0.45775862 0.45862069 0.45948276 0.46034483 0.4612069 0.46206897 0.46293103 0.4637931 0.46465517 0.46551724 0.46637931 0.46724138 0.46810345 0.46896552 0.46982759 0.47068966 0.47155172 0.47241379 0.47327586 0.47413793 0.475 0.47586207 0.47672414 0.47758621 0.47844828 0.47931034 0.48017241 0.48103448 0.48189655 0.48275862 0.48362069 0.48448276 0.48534483 0.4862069 0.48706897 0.48793103 0.4887931 0.48965517 0.49051724 0.49137931 0.49224138 0.49310345 0.49396552 0.49482759 0.49568966 0.49655172 0.49741379 0.49827586 0.49913793 0.5 0.50086207 0.50172414 0.50258621 0.50344828 0.50431034 0.50517241 0.50603448 0.50689655 0.50775862 0.50862069 0.50948276 0.51034483 0.5112069 0.51206897 0.51293103 0.5137931 0.51465517 0.51551724 0.51637931 0.51724138 0.51810345 0.51896552 0.51982759 0.52068966 0.52155172 0.52241379 0.52327586 0.52413793 0.525 0.52586207 0.52672414 0.52758621 0.52844828 0.52931034 0.53017241 0.53103448 0.53189655 0.53275862 0.53362069 0.53448276 0.53534483 0.5362069 0.53706897 0.53793103 0.5387931 0.53965517 0.54051724 0.54137931 0.54224138 0.54310345 0.54396552 0.54482759 0.54568966 0.54655172 0.54741379 0.54827586 0.54913793 0.55 0.55086207 0.55172414 0.55258621 0.55344828 0.55431034 0.55517241 0.55603448 0.55689655 0.55775862 0.55862069 0.55948276 0.56034483 0.5612069 0.56206897 0.56293103 0.5637931 0.56465517 0.56551724 0.56637931 0.56724138 0.56810345 0.56896552 0.56982759 0.57068966 0.57155172 0.57241379 0.57327586 0.57413793 0.575 0.57586207 0.57672414 0.57758621 0.57844828 0.57931034 0.58017241 0.58103448 0.58189655 0.58275862 0.58362069 0.58448276 0.58534483 0.5862069 0.58706897 0.58793103 0.5887931 0.58965517 0.59051724 0.59137931 0.59224138 0.59310345 0.59396552 0.59482759 0.59568966 0.59655172 0.59741379 0.59827586 0.59913793 0.6 0.60086207 0.60172414 0.60258621 0.60344828 0.60431034 0.60517241 0.60603448 0.60689655 0.60775862 0.60862069 0.60948276 0.61034483 0.6112069 0.61206897 0.61293103 0.6137931 0.61465517 0.61551724 0.61637931 0.61724138 0.61810345 0.61896552 0.61982759 0.62068966 0.62155172 0.62241379 0.62327586 0.62413793 0.625 0.62586207 0.62672414 0.62758621 0.62844828 0.62931034 0.63017241 0.63103448 0.63189655 0.63275862 0.63362069 0.63448276 0.63534483 0.6362069 0.63706897 0.63793103 0.6387931 0.63965517 0.64051724 0.64137931 0.64224138 0.64310345 0.64396552 0.64482759 0.64568966 0.64655172 0.64741379 0.64827586 0.64913793 0.65 0.65086207 0.65172414 0.65258621 0.65344828 0.65431034 0.65517241 0.65603448 0.65689655 0.65775862 0.65862069 0.65948276 0.66034483 0.6612069 0.66206897 0.66293103 0.6637931 0.66465517 0.66551724 0.66637931 0.66724138 0.66810345 0.66896552 0.66982759 0.67068966 0.67155172 0.67241379 0.67327586 0.67413793 0.675 0.67586207 0.67672414 0.67758621 0.67844828 0.67931034 0.68017241 0.68103448 0.68189655 0.68275862 0.68362069 0.68448276 0.68534483 0.6862069 0.68706897 0.68793103 0.6887931 0.68965517 0.69051724 0.69137931 0.69224138 0.69310345 0.69396552 0.69482759 0.69568966 0.69655172 0.69741379 0.69827586 0.69913793 0.7 0.70086207 0.70172414 0.70258621 0.70344828 0.70431034 0.70517241 0.70603448 0.70689655 0.70775862 0.70862069 0.70948276 0.71034483 0.7112069 0.71206897 0.71293103 0.7137931 0.71465517 0.71551724 0.71637931 0.71724138 0.71810345 0.71896552 0.71982759 0.72068966 0.72155172 0.72241379 0.72327586 0.72413793 0.725 0.72586207 0.72672414 0.72758621 0.72844828 0.72931034 0.73017241 0.73103448 0.73189655 0.73275862 0.73362069 0.73448276 0.73534483 0.7362069 0.73706897 0.73793103 0.7387931 0.73965517 0.74051724 0.74137931 0.74224138 0.74310345 0.74396552 0.74482759 0.74568966 0.74655172 0.74741379 0.74827586 0.74913793 0.75 0.75086207 0.75172414 0.75258621 0.75344828 0.75431034 0.75517241 0.75603448 0.75689655 0.75775862 0.75862069 0.75948276 0.76034483 0.7612069 0.76206897 0.76293103 0.7637931 0.76465517 0.76551724 0.76637931 0.76724138 0.76810345 0.76896552 0.76982759 0.77068966 0.77155172 0.77241379 0.77327586 0.77413793 0.775 0.77586207 0.77672414 0.77758621 0.77844828 0.77931034 0.78017241 0.78103448 0.78189655 0.78275862 0.78362069 0.78448276 0.78534483 0.7862069 0.78706897 0.78793103 0.7887931 0.78965517 0.79051724 0.79137931 0.79224138 0.79310345 0.79396552 0.79482759 0.79568966 0.79655172 0.79741379 0.79827586 0.79913793 0.8 0.80086207 0.80172414 0.80258621 0.80344828 0.80431034 0.80517241 0.80603448 0.80689655 0.80775862 0.80862069 0.80948276 0.81034483 0.8112069 0.81206897 0.81293103 0.8137931 0.81465517 0.81551724 0.81637931 0.81724138 0.81810345 0.81896552 0.81982759 0.82068966 0.82155172 0.82241379 0.82327586 0.82413793 0.825 0.82586207 0.82672414 0.82758621 0.82844828 0.82931034 0.83017241 0.83103448 0.83189655 0.83275862 0.83362069 0.83448276 0.83534483 0.8362069 0.83706897 0.83793103 0.8387931 0.83965517 0.84051724 0.84137931 0.84224138 0.84310345 0.84396552 0.84482759 0.84568966 0.84655172 0.84741379 0.84827586 0.84913793 0.85 0.85086207 0.85172414 0.85258621 0.85344828 0.85431034 0.85517241 0.85603448 0.85689655 0.85775862 0.85862069 0.85948276 0.86034483 0.8612069 0.86206897 0.86293103 0.8637931 0.86465517 0.86551724 0.86637931 0.86724138 0.86810345 0.86896552 0.86982759 0.87068966 0.87155172 0.87241379 0.87327586 0.87413793 0.875 0.87586207 0.87672414 0.87758621 0.87844828 0.87931034 0.88017241 0.88103448 0.88189655 0.88275862 0.88362069 0.88448276 0.88534483 0.8862069 0.88706897 0.88793103 0.8887931 0.88965517 0.89051724 0.89137931 0.89224138 0.89310345 0.89396552 0.89482759 0.89568966 0.89655172 0.89741379 0.89827586 0.89913793 0.9 0.90086207 0.90172414 0.90258621 0.90344828 0.90431034 0.90517241 0.90603448 0.90689655 0.90775862 0.90862069 0.90948276 0.91034483 0.9112069 0.91206897 0.91293103 0.9137931 0.91465517 0.91551724 0.91637931 0.91724138 0.91810345 0.91896552 0.91982759 0.92068966 0.92155172 0.92241379 0.92327586 0.92413793 0.925 0.92586207 0.92672414 0.92758621 0.92844828 0.92931034 0.93017241 0.93103448 0.93189655 0.93275862 0.93362069 0.93448276 0.93534483 0.9362069 0.93706897 0.93793103 0.9387931 0.93965517 0.94051724 0.94137931 0.94224138 0.94310345 0.94396552 0.94482759 0.94568966 0.94655172 0.94741379 0.94827586 0.94913793 0.95 0.95086207 0.95172414 0.95258621 0.95344828 0.95431034 0.95517241 0.95603448 0.95689655 0.95775862 0.95862069 0.95948276 0.96034483 0.9612069 0.96206897 0.96293103 0.9637931 0.96465517 0.96551724 0.96637931 0.96724138 0.96810345 0.96896552 0.96982759 0.97068966 0.97155172 0.97241379 0.97327586 0.97413793 0.975 0.97586207 0.97672414 0.97758621 0.97844828 0.97931034 0.98017241 0.98103448 0.98189655 0.98275862 0.98362069 0.98448276 0.98534483 0.9862069 0.98706897 0.98793103 0.9887931 0.98965517 0.99051724 0.99137931 0.99224138 0.99310345 0.99396552 0.99482759 0.99568966 0.99655172 0.99741379 0.99827586 0.99913793 1 1 1 1 1 1
  point P0 (211.8424, -56.5148)
  point P1 (210.1321, -54.9526)
  point P2 (207.6441, -52.5158)
  point P3 (204.4702, -49.5183)
  point P4 (200.4841, -46.1824)
  point P5 (195.5609, -42.5107)
  point P6 (189.7478, -38.4456)
  point P7 (183.1571, -34.0106)
  point P8 (175.8906, -29.2645)
  point P9 (168.056, -24.2847)
  point P10 (159.7583, -19.1646)
  point P11 (151.0994, -14.0012)
  point P12 (142.1777, -8.9027)
  point P13 (133.0892, -3.9852)
  point P14 (123.9205, 0.6421)
  point P15 (114.7443, 4.8464)
  point P16 (105.5657, 8.5141)
  point P17 (96.381, 11.6184)
  point P18 (87.2277, 14.1307)
  point P19 (78.1487, 16.0254)
  point P20 (69.2118, 17.3226)
  point P21 (60.4824, 18.0561)
  point P22 (52.0507, 18.2742)
  point P23 (44.0068, 18.0168)
  point P24 (36.439, 17.3186)
  point P25 (29.4262, 16.2199)
  point P26 (23.0335, 14.7625)
  point P27 (17.3284, 12.9949)
  point P28 (12.3606, 10.9678)
  point P29 (8.1759, 8.7428)
  point P30 (4.8086, 6.3877)
  point P31 (2.2948, 3.9847)
  point P32 (0.648, 1.6322)
  point P33 (-0.1128, -0.6135)
  point P34 (-0.1417, -1.0006)
  point P35 (-0.1286, -1.3705)
  point P36 (-0.108, -1.5466)
  point P37 (-0.0732, -1.7139)
  point P38 (-0.0229, -1.8752)
  point P39 (0.0484, -2.0279)
  point P40 (0.1395, -2.1833)
  point P41 (0.2458, -2.3419)